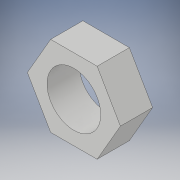
# Autodesk Inventor part: Piston nut
Saved by Autodesk Inventor 2018 (Build 220112000, 112)
## iProperties
Created: 2019-01-25
Part Number: Piston nut
Material: Generic
Document SubType Name: Modeling
Designer: s-2512711
Density: 1 g/cm^3
Appearance: Default
Author: s-2512711
Autodesk Inventor part; units mm, degrees
ref_plane "YZ Plane" through (0, 0, 0) normal (1, 0, 0) x (0, 1, 0)
ref_plane "XZ Plane" through (0, 0, 0) normal (0, 1, 0) x (-1, 0, 0)
ref_plane "XY Plane" through (0, 0, 0) normal (0, 0, 1) x (1, 0, 0)
sketch "Sketch1" plane through (0, 0, 0) normal (0, 0, 1) x (1, 0, 0)
  line L0 (13.7482, 0) -> (6.8741, -11.9062)
  line L1 (6.8741, -11.9062) -> (-6.8741, -11.9062)
  line L2 (-6.8741, -11.9062) -> (-13.7482, 0)
  line L3 (-13.7482, 0) -> (-6.8741, 11.9062)
  line L4 (-6.8741, 11.9062) -> (6.8741, 11.9063)
  line L5 (6.8741, 11.9063) -> (13.7482, 0)
  circle A0 centre (0, 0) radius 7.9375
  dimension "d0" = 23.8125
  dimension "d1" = 15.875
  constraints: 12 end point, 2 coincident, 1 centre point, 13 other
  measures "d0" distance between parallel lines of L4 L1
  measures "d1" diameter of A0
extrude "Extrusion1" add sketch "Sketch1" along normal blind 9.525
body "Solid1"
